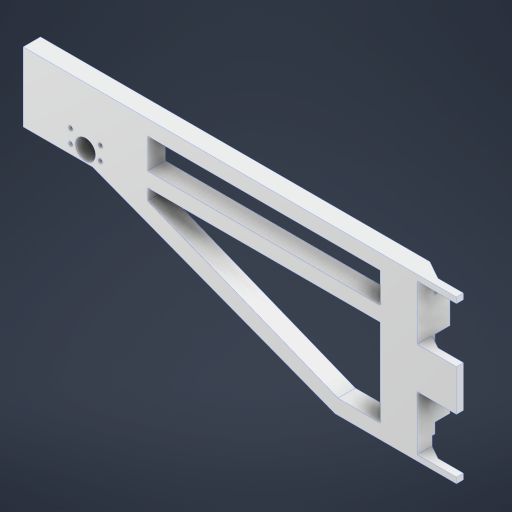
# Autodesk Inventor part: PortalFlanec
Saved by Autodesk Inventor 2024 (Build 280153000, 153)
## iProperties
Created: 2023-01-08
Part Number: PortalFlanec
Material: Aluminum 6061
Document SubType Name: Modeling
Designer: KirikDK
Density: 2.7 g/cm^3
Appearance: Aluminum - Flat
Mass: 6490.63 g
Surface Area: 3126.69 cm^2
Volume: 2403.94 cm^3
Author: KirikDK
Autodesk Inventor part; units mm, degrees
ref_plane "YZ Plane" through (0, 0, 0) normal (1, 0, 0) x (0, 1, 0)
ref_plane "XZ Plane" through (0, 0, 0) normal (0, 1, 0) x (-1, 0, 0)
ref_plane "XY Plane" through (0, 0, 0) normal (0, 0, 1) x (1, 0, 0)
sketch "Эскиз1" plane through (0, 0, 0) normal (0, 1, 0) x (-1, 0, 0)
  line L0 (650, 20) -> (0, 20)
  line L1 (0, 20) -> (0, 0)
  line L2 (0, 0) -> (650, 0)
  line L3 (650, 0) -> (650, 20)
  line L4 (650, 30) -> (0, 30)
  line L5 (0, 30) -> (0, 20)
  line L6 (0, 20) -> (650, 20)
  line L7 (650, 20) -> (650, 30)
  line L8 (0, 30) -> (0, 30)
  line L9 (0, 30) -> (0, 25.5)
  line L10 (0, 25.5) -> (0, 25.5)
  line L11 (0, 25.5) -> (0, 30)
  point P0 (0, 25.5)
  point P1 (0, 25.5)
  dimension "d0" = 20
  dimension "d1" = 10
  dimension "d2" = 650
  dimension "d3" = 650
  dimension "d4" = 0
  constraints: 24 end point, 6 equal length, 3 horizontal, 3 perpendicular
  measures "d0" distance of L0.end L1.end
  measures "d1" distance between parallel lines of L6 L4
  measures "d2" distance between parallel lines of L1 L3
  measures "d3" distance between parallel lines of L5 L7
  measures "d4" distance between parallel lines of L5 L9
extrude "Выдавливание1" add sketch "Эскиз1" along normal blind 280
sketch "Эскиз2" plane through (-650, 0, 30) normal (0, 0, 1) x (1, 0, 0)
  line L0 (-20, 160) -> (120, 160)
  line L1 (120, 160) -> (540, 0)
  line L2 (650, 0) -> (0, 0) projected
  line L3 (-20, 160) -> (-20, -90)
  line L4 (-20, -90) -> (540, -90)
  line L5 (540, -90) -> (540, 0)
  line L6 (650, 280) -> (0, 280) projected
  line L7 (0, 0) -> (0, 280) projected
  dimension "d9" = 120
  dimension "d10" = 120
  constraints: 10 end point, 2 perpendicular, 1 horizontal, 1 point on line, 1 vertical
  measures "d9" distance between parallel lines of L6 L0
  measures "d10" distance from line of L7 L0.end
extrude "Выдавливание2" cut sketch "Эскиз2" against normal blind 99
sketch "Эскиз4" plane through (0, 280, 0) normal (0, 0, -1) x (-1, 0, 0)
  line L0 (516.25, -104.25) -> (516.25, -80.75)
  line L1 (516.25, -80.75) -> (567.75, -80.75)
  line L2 (567.75, -80.75) -> (567.75, -104.25)
  line L3 (567.75, -104.25) -> (516.25, -104.25)
  line L4 (558, -120) -> (563, -120)
  line L5 (563, -120) -> (563, -113.5)
  line L6 (563, -113.5) -> (577, -113.5)
  line L7 (577, -113.5) -> (577, -71.5)
  line L8 (577, -71.5) -> (507, -71.5)
  line L9 (507, -71.5) -> (507, -113.5)
  line L10 (507, -113.5) -> (521, -113.5)
  line L11 (521, -113.5) -> (521, -120)
  line L12 (521, -120) -> (526, -120)
  line L13 (526, -120) -> (526, -108.5)
  line L14 (526, -108.5) -> (512, -108.5)
  arc A0 (512, -102.5) -> (512, -108.5) centre (512, -105.5) ccw
  line L15 (512, -102.5) -> (512, -82.5)
  arc A1 (512, -76.5) -> (512, -82.5) centre (512, -79.5) ccw
  line L16 (512, -76.5) -> (572, -76.5)
  arc A2 (572, -82.5) -> (572, -76.5) centre (572, -79.5) ccw
  line L17 (572, -82.5) -> (572, -102.5)
  arc A3 (572, -108.5) -> (572, -102.5) centre (572, -105.5) ccw
  line L18 (572, -108.5) -> (558, -108.5)
  line L19 (558, -108.5) -> (558, -120)
  circle A4 centre (516.25, -104.25) radius 3.25
  circle A5 centre (516.25, -80.75) radius 3.25
  circle A6 centre (567.75, -80.75) radius 3.25
  circle A7 centre (567.75, -104.25) radius 3.25
  circle A8 centre (542, -99.75) radius 17
  point P0 (0, -280)
  point P1 (562, -95.5)
  dimension "d11" = 4.25
  dimension "d12" = 4.25
  dimension "d13" = 4.25
  dimension "d14" = 4.25
  dimension "d15" = 19
  dimension "d16" = 34
  constraints: 38 end point, 9 centre point, 8 point on circle, 4 coincident, 2 parallel, 1 horizontal alignment, 1 perpendicular, 2 other
  measures "d11" distance between parallel lines of L15 L0
  measures "d12" distance between parallel lines of L17 L2
  measures "d14" distance between parallel lines of L18 L3
  measures "d15" distance from line of L1 A8.centre
  measures "d16" diameter of A8
sketch "Эскиз5" plane through (0, 280, 0) normal (0, 0, -1) x (-1, 0, 0)
  circle A0 centre (542, -99.75) radius 17
  line L0 (516.25, -80.75) -> (567.75, -80.75)
  line L1 (567.75, -104.25) -> (516.25, -104.25)
  line L2 (512, -76.5) -> (572, -76.5)
  line L3 (577, -71.5) -> (507, -71.5)
  line L4 (567.75, -80.75) -> (567.75, -104.25)
  line L5 (516.25, -104.25) -> (516.25, -80.75)
  circle A1 centre (516.25, -80.75) radius 3.25
  circle A2 centre (516.25, -104.25) radius 3.25
  line L6 (526, -120) -> (526, -108.5)
  line L7 (521, -113.5) -> (521, -120)
  line L8 (521, -120) -> (526, -120)
  line L9 (526, -108.5) -> (512, -108.5)
  arc A3 (512, -102.5) -> (512, -108.5) centre (512, -105.5) ccw
  line L10 (507, -113.5) -> (521, -113.5)
  line L11 (507, -71.5) -> (507, -113.5)
  line L12 (512, -102.5) -> (512, -82.5)
  arc A4 (512, -76.5) -> (512, -82.5) centre (512, -79.5) ccw
  arc A5 (572, -82.5) -> (572, -76.5) centre (572, -79.5) ccw
  circle A6 centre (567.75, -80.75) radius 3.25
  line L13 (577, -113.5) -> (577, -71.5)
  line L14 (572, -82.5) -> (572, -102.5)
  line L15 (558, -108.5) -> (558, -120)
  circle A7 centre (567.75, -104.25) radius 3.25
  line L16 (558, -120) -> (563, -120)
  line L17 (572, -108.5) -> (558, -108.5)
  arc A8 (572, -108.5) -> (572, -102.5) centre (572, -105.5) ccw
  line L18 (563, -113.5) -> (577, -113.5)
  line L19 (563, -120) -> (563, -113.5)
  point P0 (0, -280)
  point P1 (562, -95.5)
  dimension "d8" = 0
  dimension "d17" = 4.25
  dimension "d18" = 4.25
  dimension "d19" = 4.25
  dimension "d20" = 4.25
  dimension "d21" = 19
  dimension "d22" = 34
  constraints: 40 end point, 9 centre point, 8 point on circle, 4 coincident, 2 parallel, 1 perpendicular
  measures "d17" distance between parallel lines of L12 L5
  measures "d18" distance between parallel lines of L14 L4
  measures "d19" distance between parallel lines of L2 L0
  measures "d20" distance between parallel lines of L17 L1
  measures "d21" distance from line of L0 A0.centre
  measures "d22" diameter of A0
extrude "Выдавливание3" cut sketch "Эскиз4" against normal blind 55 contours L3 A4 L0 | L0 A4 L3 | A5 L1 L0 | L0 L1 A5 | A8 L3 | L3 A8 | A6 L2 L1 | L1 L2 A6 | A7 L2 L3 | L3 L2 A7
extrude "Выдавливание4" add sketch "Эскиз5" along normal blind 5 contours A4 L12 A3 L9 L6 L8 L7 L10 L11 L3 L13 L18 L19 L16 L15 L17 A8 L14 A5 L2
fillet "Сопряжение1" radius 3 2 edges at (-558, 171.5, -2.5) (-526, 171.5, -2.5)
sketch "Эскиз6" plane through (0, 280, 0) normal (0, 0, -1) x (-1, 0, 0)
  line L0 (434, -122.4) -> (105, -254)
  line L1 (105, -254) -> (105, -26)
  line L2 (105, -26) -> (434, -26)
  line L3 (434, -26) -> (434, -122.4)
  line L4 (460, -103.6971) -> (21.7305, -103.6971)
  line L5 (21.7305, -103.6971) -> (21.7305, -77.6971)
  line L6 (21.7305, -77.6971) -> (460, -77.6971)
  line L7 (460, -77.6971) -> (460, -103.6971)
  line L8 (0, 0) -> (650, 0) projected
  line L9 (105, -26) -> (32, -26)
  line L10 (32, -26) -> (32, -254)
  line L11 (32, -254) -> (105, -254)
  line L12 (105, -254) -> (105, -26)
  line L13 (507, -71.5) -> (507, -113.5) projected
  point P0 (0, -280)
  point P1 (105, -77.6971)
  point P2 (434, -77.6971)
  point P3 (440, -120)
  point P4 (105, -103.6971)
  point P5 (434, -103.6971)
  point P6 (434, -59)
  point P7 (157, -26)
  point P8 (32, -103.6971)
  point P9 (32, -77.6971)
  dimension "d54" = 26
  dimension "d55" = 26
  dimension "d68" = 73
  constraints: 24 end point, 4 parallel, 4 perpendicular, 2 horizontal, 2 point on line, 1 vertical
  measures "d54" distance between parallel lines of L8 L2
  measures "d55" distance of L4.end L5.end
  measures "d68" distance between parallel lines of L3 L13
extrude "Выдавливание5" cut sketch "Эскиз6" against normal blind 100 contours L0 L1 L4 L3 | L11 L10 L4 L1 | L6 L1 L2 L3 | L6 L10 L9 L1
sketch "Sketch14" plane through (0, 280, 0) normal (0, 0, -1) x (-1, 0, 0)
  line L0 (577, -71.5) -> (577, -113.5) projected
  line L1 (577, -77.6971) -> (629, -77.6971)
  line L2 (629, -77.6971) -> (629, -20)
  line L3 (629, -20) -> (455, -20)
  line L4 (455, -20) -> (455, -77.6971)
  line L5 (455, -77.6971) -> (507, -77.6971)
  line L6 (507, -113.5) -> (507, -71.5) projected
  line L7 (577, -77.6971) -> (577, -71.5)
  line L8 (507, -71.5) -> (577, -71.5) projected
  line L9 (507, -71.5) -> (507, -77.6971)
  line L10 (434, -77.6971) -> (32, -77.6971) projected
  point P0 (0, -280)
  dimension "d58" = 0
  dimension "d69" = 52
  dimension "d70" = 52
  constraints: 14 end point, 4 perpendicular, 4 point on line, 1 collinear, 1 horizontal
  measures "d58" distance between parallel lines of L10 L5
  measures "d69" distance between parallel lines of L2 L0
  measures "d70" distance between parallel lines of L4 L6
extrude "Extrusion13" cut sketch "Sketch14" against normal blind 20
sketch "Sketch16" plane through (-650, 280, 30) normal (0, 0, 1) x (1, 0, 0)
  line L0 (120, -120) -> (540, -280) projected
  line L1 (545, -254) -> (216, -122.4) projected
  line L2 (540, -280) -> (650, -280) projected
  line L3 (618, -254) -> (545, -254) projected
  line L4 (618, -103.6971) -> (618, -254) projected
  line L5 (650, -280) -> (650, 0) projected
  line L6 (216, -103.6971) -> (618, -103.6971) projected
  line L7 (618, -77.6971) -> (216, -77.6971) projected
  line L8 (216, -26) -> (618, -26) projected
  line L9 (618, -26) -> (618, -77.6971) projected
  line L10 (0, 0) -> (650, 0) projected
  line L11 (216, -77.6971) -> (216, -26) projected
  line L12 (0, -120) -> (120, -120) projected
  line L13 (0, -120) -> (0, 0) projected
  circle A0 centre (82.25, -80.75) radius 3.25 projected
  circle A1 centre (82.25, -104.25) radius 3.25 projected
  circle A2 centre (108, -99.75) radius 17 projected
  circle A3 centre (133.75, -104.25) radius 3.25 projected
  circle A4 centre (133.75, -80.75) radius 3.25 projected
sketch "Sketch17" plane through (0, 0, 30) normal (1, 0, 0) x (0, 0, -1)
  line L0 (0, 175.6551) -> (30, 175.6551)
  line L1 (30, 175.6551) -> (30, 104)
  line L2 (30, 104) -> (0, 104)
  line L3 (0, 104) -> (0, 175.6551)
  line L4 (30, 26) -> (0, 26) projected
  line L5 (0, 26) -> (30, 26)
  line L6 (30, 26) -> (30, 0)
  line L7 (30, 0) -> (0, 0)
  line L8 (0, 0) -> (0, 26)
  line L9 (30, 0) -> (30, 280) projected
  line L10 (0, 253.6551) -> (30, 253.6551)
  line L11 (30, 253.6551) -> (30, 280)
  line L12 (30, 280) -> (0, 280)
  line L13 (0, 280) -> (0, 253.6551)
  dimension "d61" = 26.345
  dimension "d73" = 78
  dimension "d74" = 78
  constraints: 24 end point, 6 parallel, 3 horizontal, 3 perpendicular
  measures "d61" distance of L12.end L10.start
  measures "d73" distance between parallel lines of L10 L0
  measures "d74" distance between parallel lines of L2 L5
extrude "Extrusion14" add sketch "Sketch17" along normal blind 100
sketch "Sketch18" plane through (-650, 160, 30) normal (0, 0, 1) x (1, 0, 0)
  line L0 (650, 15.6551) -> (750, 15.6551) projected
  line L1 (750, 15.6551) -> (682.7907, 15.6551)
  line L2 (682.7907, 15.6551) -> (682.7907, 110)
  line L3 (682.7907, 110) -> (750, 110)
  line L4 (750, 110) -> (750, 15.6551)
  line L5 (650, -56) -> (750, -56) projected
  line L6 (750, -56) -> (682.7907, -56)
  line L7 (682.7907, -56) -> (682.7907, -150)
  line L8 (682.7907, -150) -> (750, -150)
  line L9 (750, -150) -> (750, -56)
  line L10 (0, 120) -> (750, 120) projected
  line L11 (540, -160) -> (750, -160) projected
  point P0 (650, -160)
  point P1 (682.7907, -56)
  point P2 (682.7907, 15.6551)
  dimension "d64" = 10
  dimension "d65" = 10
  constraints: 16 end point, 4 parallel, 2 horizontal, 2 perpendicular, 1 point on line
  measures "d64" distance between parallel lines of L3 L10
  measures "d65" distance between parallel lines of L8 L11
extrude "Extrusion15" cut sketch "Sketch18" against normal blind 30
sketch "Sketch19" plane through (0, 280, 0) normal (0, 1, 0) x (1, 0, 0)
  line L0 (100, -30) -> (100, 0) projected
  line L1 (100, -9) -> (100, -9)
  line L2 (100, -9) -> (100, -18)
  line L3 (100, -18) -> (56, -18)
  line L4 (56, -18) -> (6, 10)
  line L5 (6, 10) -> (100, 10)
  line L6 (100, 10) -> (100, -9)
  point P0 (0, 0)
  dimension "d75" = 0
  dimension "d76" = 0
  dimension "d77" = 19
  dimension "d79" = 94
  dimension "d80" = 50
  constraints: 12 end point, 2 parallel, 1 horizontal, 1 perpendicular, 1 point on line
  measures "d75" distance of L1.start L1.end
  measures "d76" horizontal distance of L1.start L2.end
  measures "d77" distance of L5.end L1.start
  measures "d79" distance of L4.end L5.end
  measures "d80" horizontal distance of L4.end L3.end
extrude "Extrusion16" cut sketch "Sketch19" against normal blind 1000
sketch "Sketch20" plane through (-650, 160, 0) normal (0, 0, -1) x (-1, 0, 0)
  line L0 (-650, -134) -> (-650, -56) projected
  line L1 (-650, 93.6551) -> (-682.7907, 93.6551) projected
  line L2 (-650, -134) -> (-682.7907, -134)
  line L3 (-682.7907, -134) -> (-682.7907, 93.6551)
  line L4 (-682.7907, 93.6551) -> (-650, 93.6551)
  line L5 (-650, 93.6551) -> (-650, -134)
  point P0 (-650, -160)
  constraints: 8 end point, 2 parallel, 1 horizontal, 1 perpendicular
extrude "Extrusion17" add sketch "Sketch20" against normal up to surface (30 mm away)
sketch "Sketch21" plane through (-650, 160, 0) normal (0, 0, -1) x (-1, 0, 0)
  line L0 (-682.7907, 93.6551) -> (-682.7907, -134) projected
  line L1 (-682.7907, -56) -> (-627.7907, -56)
  line L2 (-627.7907, -56) -> (-627.7907, -116)
  line L3 (-627.7907, -116) -> (-682.7907, -116)
  line L4 (-682.7907, -116) -> (-682.7907, -56)
  line L5 (-706, 15.6551) -> (-682.7907, 15.6551) projected
  line L6 (-682.7907, 15.6551) -> (-627.7907, 15.6551)
  line L7 (-627.7907, 15.6551) -> (-627.7907, 75.6551)
  line L8 (-627.7907, 75.6551) -> (-682.7907, 75.6551)
  line L9 (-682.7907, 75.6551) -> (-682.7907, 15.6551)
  point P0 (-650, -160)
  dimension "d83" = 55
  dimension "d84" = 55
  dimension "d85" = 60
  dimension "d86" = 60
  constraints: 16 end point, 4 parallel, 2 horizontal, 2 perpendicular, 1 point on line
  measures "d83" distance of L1.start L1.end
  measures "d84" distance of L5.end L6.end
  measures "d85" distance of L1.end L2.end
  measures "d86" distance of L6.end L7.end
extrude "Extrusion18" add sketch "Sketch21" along normal blind 26
